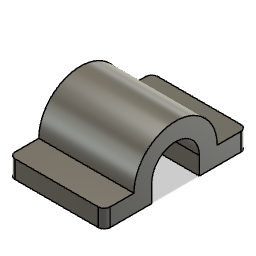
Modify 3 (Autodesk Fusion 360 design; units mm, degrees)
Autodesk Fusion 360 part; units mm, degrees
sketch "Sketch1" plane through (0, 0, 0) normal (1, 0, 0) x (0, 0, -1)
  line L0 (20, 0) -> (60, 0)
  line L1 (-20, 0) -> (-60, 0)
  line L2 (-60, 0) -> (-60, 15)
  line L3 (60, 0) -> (60, 15)
  arc A0 (35, 15) -> (-35, 15) centre (0, 15) ccw
  arc A1 (20, 15) -> (-20, 15) centre (0, 15) ccw
  line L4 (20, 15) -> (20, 0)
  line L5 (-20, 15) -> (-20, 0)
  line L6 (-60, 15) -> (-35, 15)
  line L7 (35, 15) -> (60, 15)
  dimension "d1" = 60
  dimension "d2" = 60
  dimension "d3" = 15
  dimension "d4" = 15
  constraint horizontal L0
  constraint parallel L0 L1
  constraint perpendicular L1 L2
  constraint perpendicular L0 L3
  constraint concentric A0 A1
  constraint coincident A1.start L6
  constraint coincident A0.start L6
  constraint tangent A1 L4
  constraint tangent A1 L5
  constraint collinear L6 L7
  constraint coincident A0.centre L6
  measures "d1" distance of origin L0.end
  measures "d2" distance of origin L1.end
  measures "d3" distance of L1.end L2.end
  measures "d4" distance of L0.end L3.end
extrude "Extrude1" add sketch "Sketch1" along normal blind 80
fillet "Fillet1" radius 5 4 edges at (0, 7.5, 60) (80, 7.5, 60) (80, 7.5, -60) (0, 7.5, -60)
